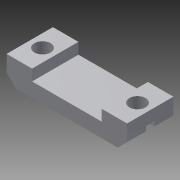
# Autodesk Inventor part: LCDDerivativeStrainRelief
Saved by Autodesk Inventor 2015 SP1 (Build 190203100, 203)
## iProperties
Created: 2015-04-17
Part Number: LCDDerivativeStrainRelief
Material: ABS Plastic
Document SubType Name: Modeling
Designer: Jack
Density: 1.06 g/cm^3
Appearance: Smooth - White
Author: Jack
Autodesk Inventor part; units mm, degrees
ref_plane "YZ Plane" through (0, 0, 0) normal (1, 0, 0) x (0, 1, 0)
ref_plane "XZ Plane" through (0, 0, 0) normal (0, 1, 0) x (-1, 0, 0)
ref_plane "XY Plane" through (0, 0, 0) normal (0, 0, 1) x (1, 0, 0)
sketch "Sketch1" plane through (0, 0, 0) normal (0, 0, 1) x (1, 0, 0)
  line L0 (0, 0) -> (26, 0)
  line L1 (26, 0) -> (26, 10)
  line L2 (26, 10) -> (0, 10)
  line L3 (0, 10) -> (0, 0)
  dimension "d0" = 26
  dimension "d1" = 10
  constraints: 8 end point, 2 parallel, 1 horizontal, 1 perpendicular
  measures "d0" distance of L1.end L2.end
  measures "d1" distance of L2.end L0.start
extrude "Extrusion1" add sketch "Sketch1" along normal blind 5.5
sketch "Sketch2" plane through (0, 10, 0) normal (0, 1, 0) x (1, 0, 0)
  line L0 (26, -5.5) -> (0, -5.5) projected
  line L1 (26, 0) -> (26, -5.5) projected
  line L2 (5.5, -5.5) -> (5.5, -3.1)
  line L3 (5.5, -3.1) -> (20.5, -3.1)
  line L4 (20.5, -3.1) -> (20.5, -5.5)
  dimension "d4" = 15
  dimension "d5" = 2.4
  dimension "d6" = 5.5
  constraints: 6 end point, 2 perpendicular, 2 point on line, 1 vertical
  measures "d4" distance of L2.end L3.end
  measures "d5" distance of L3.end L4.end
  measures "d6" distance between parallel lines of L1 L4
extrude "Extrusion2" cut sketch "Sketch2" against normal up to next
chamfer "Chamfer1" distance 2 angle 45 2 edges at (0, 5, 0) (26, 5, 0)
sketch "Sketch3" plane through (0, 0, 0) normal (0, 0, -1) x (-1, 0, 0)
  line L0 (-2, 0) -> (-24, 0) projected
  line L1 (-2, 0) -> (0, 0) projected
  line L2 (0, 0) -> (0, 10) projected
  line L3 (0, 10) -> (-2, 10) projected
  line L4 (-2, 10) -> (-2, 0) projected
  line L5 (-24, 10) -> (-26, 10) projected
  line L6 (-26, 10) -> (-26, 0) projected
  line L7 (-26, 0) -> (-24, 0) projected
  line L8 (-24, 0) -> (-24, 10) projected
  point P0 (-2.75, 5)
  point P1 (-23.25, 5)
  dimension "d12" = 2.75
  dimension "d13" = 2.75
  dimension "d14" = 5
  constraints: 1 horizontal alignment
  measures "d12" distance from line of L6 point (-23.25, 5)
  measures "d13" distance from line of point (-2.75, 5) L2
  measures "d14" distance from line of L0 point (-23.25, 5)
hole "Hole1" at (2.75, 5, 0) at (23.25, 5, 0) direction (0, 0, 1) diameter 3.5 depth 8 tip angle 118 counterbore diameter 5.8 counterbore depth 3
body "Solid1"
